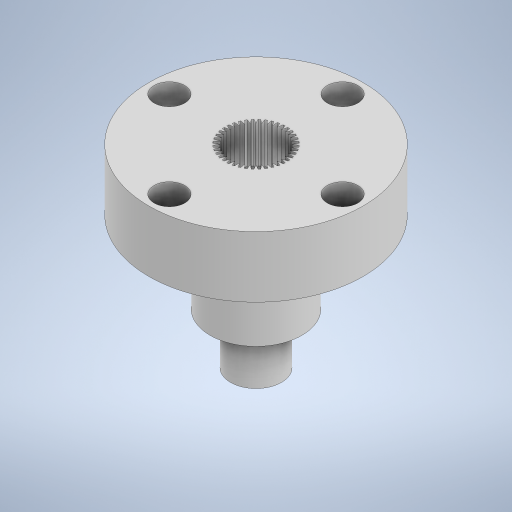
# Autodesk Inventor part: spinner
Saved by Autodesk Inventor 2024 (Build 280153000, 153)
## iProperties
Created: 2024-09-30
Part Number: spinner
Material: Generic
Document SubType Name: Modeling
Designer: m_kni
Density: 1 g/cm^3
Appearance: Default
Author: m_kni
Autodesk Inventor part; units mm, degrees
ref_plane "YZ Plane" through (0, 0, 0) normal (1, 0, 0) x (0, 1, 0)
ref_plane "XZ Plane" through (0, 0, 0) normal (0, 1, 0) x (-1, 0, 0)
ref_plane "XY Plane" through (0, 0, 0) normal (0, 0, 1) x (1, 0, 0)
sketch "Sketch1" plane through (0, 0, 0) normal (0, 1, 0) x (-1, 0, 0)
  line L0 (-12.7, 12.7) -> (12.7, 12.7)
  line L1 (12.7, 12.7) -> (12.7, -12.7)
  line L2 (12.7, -12.7) -> (-12.7, -12.7)
  line L3 (-12.7, -12.7) -> (-12.7, 12.7)
  line L4 (-12.7, 12.7) -> (12.7, -12.7) construction
  line L5 (12.7, 12.7) -> (-12.7, -12.7) construction
  line L6 (-11.4786, 11.4786) -> (11.4786, 11.4786)
  line L7 (11.4786, 11.4786) -> (11.4786, -11.4786)
  line L8 (11.4786, -11.4786) -> (-11.4786, -11.4786)
  line L9 (-11.4786, -11.4786) -> (-11.4786, 11.4786)
  line L10 (-11.4786, 11.4786) -> (11.4786, -11.4786) construction
  line L11 (11.4786, 11.4786) -> (-11.4786, -11.4786) construction
  line L12 (-25.4, -25.4) -> (25.4, -25.4)
  line L13 (25.4, -25.4) -> (25.4, 25.4)
  line L14 (25.4, 25.4) -> (-25.4, 25.4)
  line L15 (-25.4, 25.4) -> (-25.4, -25.4)
  line L16 (-25.4, -25.4) -> (25.4, 25.4) construction
  line L17 (25.4, -25.4) -> (-25.4, 25.4) construction
  circle A0 centre (0, 0) radius 5.5
  circle A1 centre (11.4786, 11.4786) radius 5.5
  circle A2 centre (11.4786, -11.4786) radius 5.5
  circle A3 centre (-11.4786, 11.4786) radius 5.5
  circle A4 centre (-11.4786, -11.4786) radius 5.5
  circle A5 centre (-25.4, 25.4) radius 5.5
  circle A6 centre (25.4, 25.4) radius 5.5
  circle A7 centre (25.4, -25.4) radius 5.5
  circle A8 centre (-25.4, -25.4) radius 5.5
  line L18 (7.5895, 15.3677) -> (21.5109, 29.2891)
  line L19 (29.2891, 21.5109) -> (15.3677, 7.5895)
  line L20 (15.3677, -7.5895) -> (29.2891, -21.5109)
  line L21 (-7.5895, -15.3677) -> (-21.5109, -29.2891)
  line L22 (-29.2891, 21.5109) -> (-15.3677, 7.5895)
  line L23 (7.5895, -15.3677) -> (21.5109, -29.2891)
  line L24 (-14.6585, -6.991) -> (-28.5798, -20.9124)
  line L25 (-8.9306, 16.3528) -> (-21.4569, 29.2343)
  line L26 (-35, -35) -> (35, -35)
  line L27 (35, -35) -> (35, 35)
  line L28 (35, 35) -> (-35, 35)
  line L29 (-35, 35) -> (-35, -35)
  line L30 (-35, -35) -> (35, 35) construction
  line L31 (35, -35) -> (-35, 35) construction
  circle A9 centre (11.4786, 11.4786) radius 2.5
  circle A10 centre (25.4, 25.4) radius 2.5
  line L32 (27.1678, 23.6322) -> (13.2464, 9.7109)
  line L33 (23.7072, 27.2397) -> (9.7111, 13.2466)
  line L34 (0, 0) -> (0, 35)
  line L35 (35, 0) -> (0, 0)
  line L36 (-27.1678, 23.6322) -> (-13.2464, 9.7109)
  circle A11 centre (-25.4, 25.4) radius 2.5
  line L37 (-23.7072, 27.2397) -> (-9.7111, 13.2466)
  circle A12 centre (-11.4786, 11.4786) radius 2.5
  circle A13 centre (25.4, -25.4) radius 2.5
  line L38 (23.7072, -27.2397) -> (9.7111, -13.2466)
  line L39 (27.1678, -23.6322) -> (13.2464, -9.7109)
  circle A14 centre (11.4786, -11.4786) radius 2.5
  circle A15 centre (-11.4786, -11.4786) radius 2.5
  line L40 (-23.7072, -27.2397) -> (-9.7111, -13.2466)
  line L41 (-27.1678, -23.6322) -> (-13.2464, -9.7109)
  line L42 (25.4, 25.4) -> (-25.4, -25.4) construction
  circle A16 centre (-25.4, -25.4) radius 2.5
  circle A17 centre (0, 0) radius 10.5
  circle A18 centre (0, 0) radius 6.5
  dimension "d0" = 25.4
  dimension "d1" = 25.4
  dimension "d2" = 50.8
  dimension "d3" = 50.8
  dimension "d4" = 11
  dimension "d5" = 11
  dimension "d6" = 11
  dimension "d7" = 11
  dimension "d8" = 11
  dimension "d9" = 11
  dimension "d10" = 11
  dimension "d11" = 11
  dimension "d12" = 11
  dimension "d13" = 70
  dimension "d14" = 5
  dimension "d15" = 5
  dimension "d16" = 21
  dimension "d17" = 13
  constraints: 86 end point, 32 point on circle, 19 centre point, 18 symmetric about line, 14 coincident, 13 tangent, 10 midpoint, 8 parallel, 5 horizontal, 5 perpendicular, 3 point on line, 6 other
  measures "d0" distance of L1.end L2.end
  measures "d1" distance of L0.end L1.end
  measures "d2" distance of L14.end L13.end
  measures "d3" distance of L13.end L12.end
  measures "d4" diameter of A0
  measures "d5" diameter of A1
  measures "d6" diameter of A2
  measures "d7" diameter of A3
  measures "d8" diameter of A4
  measures "d9" diameter of A5
  measures "d10" diameter of A6
  measures "d11" diameter of A7
  measures "d12" diameter of A8
  measures "d13" distance of L28.end L27.end
  measures "d14" diameter of A9
  measures "d15" diameter of A10
  measures "d16" diameter of A17
  measures "d17" diameter of A18
extrude "Extrusion1" add sketch "Sketch1" along normal blind 8 contours A18 L35 A0 L34 | L34 A0 L35 A18 | L34 L35 A0 | A0 L35 L34
sketch "Sketch2" plane through (0, 8, 0) normal (0, 1, 0) x (1, 0, 0)
  line L0 (-12.7, 12.7) -> (12.7, 12.7)
  line L1 (12.7, 12.7) -> (12.7, -12.7)
  line L2 (12.7, -12.7) -> (-12.7, -12.7)
  line L3 (-12.7, -12.7) -> (-12.7, 12.7)
  line L4 (-12.7, 12.7) -> (12.7, -12.7) construction
  line L5 (12.7, 12.7) -> (-12.7, -12.7) construction
  line L6 (-11.4786, 11.4786) -> (11.4786, 11.4786)
  line L7 (11.4786, 11.4786) -> (11.4786, -11.4786)
  line L8 (11.4786, -11.4786) -> (-11.4786, -11.4786)
  line L9 (-11.4786, -11.4786) -> (-11.4786, 11.4786)
  line L10 (-11.4786, 11.4786) -> (11.4786, -11.4786) construction
  line L11 (11.4786, 11.4786) -> (-11.4786, -11.4786) construction
  line L12 (-25.4, -25.4) -> (25.4, -25.4)
  line L13 (25.4, -25.4) -> (25.4, 25.4)
  line L14 (25.4, 25.4) -> (-25.4, 25.4)
  line L15 (-25.4, 25.4) -> (-25.4, -25.4)
  line L16 (-25.4, -25.4) -> (25.4, 25.4) construction
  line L17 (25.4, -25.4) -> (-25.4, 25.4) construction
  circle A0 centre (0, 0) radius 5.5
  circle A1 centre (11.4786, 11.4786) radius 5.5
  circle A2 centre (11.4786, -11.4786) radius 5.5
  circle A3 centre (-11.4786, 11.4786) radius 5.5
  circle A4 centre (-11.4786, -11.4786) radius 5.5
  circle A5 centre (-25.4, 25.4) radius 5.5
  circle A6 centre (25.4, 25.4) radius 5.5
  circle A7 centre (25.4, -25.4) radius 5.5
  circle A8 centre (-25.4, -25.4) radius 5.5
  line L18 (7.5895, 15.3677) -> (21.5109, 29.2891)
  line L19 (29.2891, 21.5109) -> (15.3677, 7.5895)
  line L20 (15.3677, -7.5895) -> (29.2891, -21.5109)
  line L21 (-7.5895, -15.3677) -> (-21.5109, -29.2891)
  line L22 (-29.2891, 21.5109) -> (-15.3677, 7.5895)
  line L23 (7.5895, -15.3677) -> (21.5109, -29.2891)
  line L24 (-16.1952, -8.6495) -> (-30.1166, -22.5709)
  line L25 (-9.6329, 16.6597) -> (-21.393, 29.1675)
  line L26 (-35, -35) -> (35, -35)
  line L27 (35, -35) -> (35, 35)
  line L28 (35, 35) -> (-35, 35)
  line L29 (-35, 35) -> (-35, -35)
  line L30 (-35, -35) -> (35, 35) construction
  line L31 (35, -35) -> (-35, 35) construction
  circle A9 centre (11.4786, 11.4786) radius 2.5
  circle A10 centre (25.4, 25.4) radius 2.5
  line L32 (27.1678, 23.6322) -> (13.2464, 9.7109)
  line L33 (23.5125, 27.0393) -> (9.7114, 13.247)
  line L34 (0, 0) -> (0, 35)
  line L35 (35, 0) -> (0, 0)
  line L36 (-27.1678, 23.6322) -> (-13.2464, 9.7109)
  circle A11 centre (-25.4, 25.4) radius 2.5
  line L37 (-23.5125, 27.0393) -> (-9.7114, 13.247)
  circle A12 centre (-11.4786, 11.4786) radius 2.5
  circle A13 centre (25.4, -25.4) radius 2.5
  line L38 (23.5125, -27.0393) -> (9.7114, -13.247)
  line L39 (27.1678, -23.6322) -> (13.2464, -9.7109)
  circle A14 centre (11.4786, -11.4786) radius 2.5
  circle A15 centre (-11.4786, -11.4786) radius 2.5
  line L40 (-23.5125, -27.0393) -> (-9.7114, -13.247)
  line L41 (-27.1678, -23.6322) -> (-13.2464, -9.7109)
  line L42 (25.4, 25.4) -> (-25.4, -25.4) construction
  circle A16 centre (-25.4, -25.4) radius 2.5
  circle A17 centre (0, 0) radius 10.5
  dimension "d20" = 25.4
  dimension "d21" = 25.4
  dimension "d22" = 50.8
  dimension "d23" = 50.8
  dimension "d24" = 11
  dimension "d25" = 11
  dimension "d26" = 11
  dimension "d27" = 11
  dimension "d28" = 11
  dimension "d29" = 11
  dimension "d30" = 11
  dimension "d31" = 11
  dimension "d32" = 11
  dimension "d33" = 70
  dimension "d34" = 5
  dimension "d35" = 5
  dimension "d36" = 21
  constraints: 86 end point, 32 point on circle, 18 centre point, 18 symmetric about line, 13 coincident, 13 tangent, 10 midpoint, 8 parallel, 5 horizontal, 5 perpendicular, 3 point on line, 6 other
  measures "d20" distance of L1.end L2.end
  measures "d21" distance of L0.end L1.end
  measures "d22" distance of L14.end L13.end
  measures "d23" distance of L13.end L12.end
  measures "d24" diameter of A0
  measures "d25" diameter of A1
  measures "d26" diameter of A2
  measures "d27" diameter of A3
  measures "d28" diameter of A4
  measures "d29" diameter of A5
  measures "d30" diameter of A6
  measures "d31" diameter of A7
  measures "d32" diameter of A8
  measures "d33" distance of L28.end L27.end
  measures "d34" diameter of A9
  measures "d35" diameter of A10
  measures "d36" diameter of A17
extrude "Extrusion2" add sketch "Sketch2" along normal blind 6 contours A17 L35 A0 L34 | L34 A0 L35 A17 | L34 L35 A0 | A0 L35 L34
sketch "Sketch3" plane through (0, 8, 0) normal (0, -1, 0) x (1, 0, 0)
  circle A0 centre (0, -8.5) radius 1.5
  circle A1 centre (8.5, 0) radius 1.5
  circle A2 centre (-8.5, 0) radius 1.5
  circle A3 centre (0, 8.5) radius 1.5
  point P0 (0, 0)
  dimension "d39" = 8.5
  dimension "d40" = 8.5
  dimension "d41" = 8.5
  dimension "d42" = 8.5
  dimension "d43" = 3
  dimension "d44" = 3
  dimension "d45" = 3
  dimension "d46" = 3
  constraints: 4 centre point, 4 coincident
  measures "d39" distance of point (0, -8.5) point (0, 0)
  measures "d40" distance of point (-8.5, 0) point (0, 0)
  measures "d41" distance of point (0, 8.5) point (0, 0)
  measures "d42" distance of point (8.5, 0) point (0, 0)
  measures "d43" diameter of A0
  measures "d44" diameter of A1
  measures "d45" diameter of A2
  measures "d46" diameter of A3
extrude "Extrusion3" cut sketch "Sketch3" against normal blind 6
sketch "Sketch4" plane through (0, 0, 0) normal (0, -1, 0) x (1, 0, 0)
  circle A0 centre (0, 0) radius 2.5
  dimension "d49" = 5
  constraints: 1 centre point, 1 coincident
  measures "d49" diameter of A0
extrude "Extrusion4" add sketch "Sketch4" along normal blind 5
sketch "Sketch5" plane through (0, 0, 0) normal (0, -1, 0) x (1, 0, 0)
  circle A0 centre (0, 0) radius 4.5
  circle A1 centre (0, 0) radius 6.5
  dimension "d52" = 9
  constraints: 2 centre point, 2 coincident
  measures "d52" diameter of A0
extrude "Extrusion5" cut sketch "Sketch5" against normal blind 12
sketch "Sketch7" plane through (0, 14, 0) normal (0, 1, 0) x (1, 0, 0)
  circle A0 centre (0, 0) radius 3
  circle A1 centre (0, 0) radius 2.5
  line L0 (0, -2.5) -> (-0.1401, -2.9967)
  line L1 (0, -2.5) -> (0.1401, -2.9967)
  line L2 (0.3911, -2.4692) -> (0.6072, -2.9379)
  line L3 (0.3911, -2.4692) -> (0.3304, -2.9817)
  line L4 (0.7725, -2.3776) -> (1.0593, -2.8068)
  line L5 (0.7725, -2.3776) -> (0.7928, -2.8933)
  line L6 (1.135, -2.2275) -> (1.4853, -2.6065)
  line L7 (1.135, -2.2275) -> (1.2357, -2.7337)
  line L8 (1.4695, -2.0225) -> (1.8748, -2.3421)
  line L9 (1.4695, -2.0225) -> (1.6481, -2.5067)
  line L10 (1.7678, -1.7678) -> (2.2181, -2.0199)
  line L11 (1.7678, -1.7678) -> (2.0199, -2.2181)
  line L12 (2.0225, -1.4695) -> (2.5067, -1.6481)
  line L13 (2.0225, -1.4695) -> (2.3421, -1.8748)
  line L14 (2.2275, -1.135) -> (2.7337, -1.2357)
  line L15 (2.2275, -1.135) -> (2.6065, -1.4853)
  line L16 (2.3776, -0.7725) -> (2.8933, -0.7928)
  line L17 (2.3776, -0.7725) -> (2.8068, -1.0593)
  line L18 (2.4692, -0.3911) -> (2.9817, -0.3304)
  line L19 (2.4692, -0.3911) -> (2.9379, -0.6072)
  line L20 (2.5, 0) -> (2.9967, 0.1401)
  line L21 (2.5, 0) -> (2.9967, -0.1401)
  line L22 (2.4692, 0.3911) -> (2.9379, 0.6072)
  line L23 (2.4692, 0.3911) -> (2.9817, 0.3304)
  line L24 (2.3776, 0.7725) -> (2.8068, 1.0593)
  line L25 (2.3776, 0.7725) -> (2.8933, 0.7928)
  line L26 (2.2275, 1.135) -> (2.6065, 1.4853)
  line L27 (2.2275, 1.135) -> (2.7337, 1.2357)
  line L28 (2.0225, 1.4695) -> (2.3421, 1.8748)
  line L29 (2.0225, 1.4695) -> (2.5067, 1.6481)
  line L30 (1.7678, 1.7678) -> (2.0199, 2.2181)
  line L31 (1.7678, 1.7678) -> (2.2181, 2.0199)
  line L32 (1.4695, 2.0225) -> (1.6481, 2.5067)
  line L33 (1.4695, 2.0225) -> (1.8748, 2.3421)
  line L34 (1.135, 2.2275) -> (1.2357, 2.7337)
  line L35 (1.135, 2.2275) -> (1.4853, 2.6065)
  line L36 (0.7725, 2.3776) -> (0.7928, 2.8933)
  line L37 (0.7725, 2.3776) -> (1.0593, 2.8068)
  line L38 (0.3911, 2.4692) -> (0.3304, 2.9817)
  line L39 (0.3911, 2.4692) -> (0.6072, 2.9379)
  line L40 (0, 2.5) -> (-0.1401, 2.9967)
  line L41 (0, 2.5) -> (0.1401, 2.9967)
  line L42 (-0.3911, 2.4692) -> (-0.6072, 2.9379)
  line L43 (-0.3911, 2.4692) -> (-0.3304, 2.9817)
  line L44 (-0.7725, 2.3776) -> (-1.0593, 2.8068)
  line L45 (-0.7725, 2.3776) -> (-0.7928, 2.8933)
  line L46 (-1.135, 2.2275) -> (-1.4853, 2.6065)
  line L47 (-1.135, 2.2275) -> (-1.2357, 2.7337)
  line L48 (-1.4695, 2.0225) -> (-1.8748, 2.3421)
  line L49 (-1.4695, 2.0225) -> (-1.6481, 2.5067)
  line L50 (-1.7678, 1.7678) -> (-2.2181, 2.0199)
  line L51 (-1.7678, 1.7678) -> (-2.0199, 2.2181)
  line L52 (-2.0225, 1.4695) -> (-2.5067, 1.6481)
  line L53 (-2.0225, 1.4695) -> (-2.3421, 1.8748)
  line L54 (-2.2275, 1.135) -> (-2.7337, 1.2357)
  line L55 (-2.2275, 1.135) -> (-2.6065, 1.4853)
  line L56 (-2.3776, 0.7725) -> (-2.8933, 0.7928)
  line L57 (-2.3776, 0.7725) -> (-2.8068, 1.0593)
  line L58 (-2.4692, 0.3911) -> (-2.9817, 0.3304)
  line L59 (-2.4692, 0.3911) -> (-2.9379, 0.6072)
  line L60 (-2.5, 0) -> (-2.9967, -0.1401)
  line L61 (-2.5, 0) -> (-2.9967, 0.1401)
  line L62 (-2.4692, -0.3911) -> (-2.9379, -0.6072)
  line L63 (-2.4692, -0.3911) -> (-2.9817, -0.3304)
  line L64 (-2.3776, -0.7725) -> (-2.8068, -1.0593)
  line L65 (-2.3776, -0.7725) -> (-2.8933, -0.7928)
  line L66 (-2.2275, -1.135) -> (-2.6065, -1.4853)
  line L67 (-2.2275, -1.135) -> (-2.7337, -1.2357)
  line L68 (-2.0225, -1.4695) -> (-2.3421, -1.8748)
  line L69 (-2.0225, -1.4695) -> (-2.5067, -1.6481)
  line L70 (-1.7678, -1.7678) -> (-2.0199, -2.2181)
  line L71 (-1.7678, -1.7678) -> (-2.2181, -2.0199)
  line L72 (-1.4695, -2.0225) -> (-1.6481, -2.5067)
  line L73 (-1.4695, -2.0225) -> (-1.8748, -2.3421)
  line L74 (-1.135, -2.2275) -> (-1.2357, -2.7337)
  line L75 (-1.135, -2.2275) -> (-1.4853, -2.6065)
  line L76 (-0.7725, -2.3776) -> (-0.7928, -2.8933)
  line L77 (-0.7725, -2.3776) -> (-1.0593, -2.8068)
  line L78 (-0.3911, -2.4692) -> (-0.3304, -2.9817)
  line L79 (-0.3911, -2.4692) -> (-0.6072, -2.9379)
  dimension "d58" = 6
  dimension "d59" = 5
  dimension "d63" = 360
  constraints: 160 end point, 2 coincident, 1 vertical alignment, 205 other
extrude "Extrusion6" cut sketch "Sketch7" against normal blind 4 contours L20 A1 L23 A0 | A0 L18 A1 L21 | A1 | L22 A1 L25 A0 | L19 A0 L16 A1 | A1 L27 A0 L24 | L17 A0 L14 A1 | A1 L29 A0 L26 | L15 A0 L12 A1 | A1 L31 A0 L28 | L13 A0 L10 A1 | A1 L33 A0 L30 | L11 A0 L8 A1 | A1 L35 A0 L32 | L9 A0 L6 A1 | A1 L37 A0 L34 | L7 A0 L4 A1 | A1 L39 A0 L36 | L5 A0 L2 A1 | A1 L41 A0 L38 | L3 A0 L1 A1 | A1 L43 A0 L40 | L0 A0 L78 A1 | A1 L45 A0 L42 | L79 A0 L76 A1 | A1 L47 A0 L44 | L77 A0 L74 A1 | A1 L49 A0 L46 | L75 A0 L72 A1 | A1 L51 A0 L48 | L73 A0 L70 A1 | A1 L53 A0 L50 | L71 A0 L68 A1 | A1 L55 A0 L52 | L69 A0 L66 A1 | A1 L57 A0 L54 | L67 A0 L64 A1 | A1 L59 A0 L56 | L65 A0 L62 A1 | A1 L61 A0 L58 | L63 A0 L60 A1
body "Solid1"
